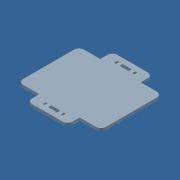
# Autodesk Inventor part: base protopress
Saved by Autodesk Inventor 2014 (Build 180170000, 170)
## iProperties
Created: 2013-09-11
Part Number: base protopress
Material: Glass
Document SubType Name: Modeling
Designer: Lefo
Density: 2.18 g/cm^3
Appearance: Clear
Author: Lefo
Autodesk Inventor part; units mm, degrees
ref_plane "YZ Plane" through (0, 0, 0) normal (1, 0, 0) x (0, 1, 0)
ref_plane "XZ Plane" through (0, 0, 0) normal (0, 1, 0) x (-1, 0, 0)
sketch "Sketch1" plane through (0, 0, 0) normal (0, 1, 0) x (-1, 0, 0)
  line L0 (0, 0) -> (-82, 0)
  line L1 (-82, 0) -> (-82, 60.3)
  line L2 (-82, 60.3) -> (0, 60.3)
  line L3 (0, 60.3) -> (0, 0)
  dimension "d0" = 82
  dimension "d1" = 60.3
  constraints: 8 end point, 2 parallel, 1 horizontal, 1 perpendicular
  measures "d0" distance of L1.end L2.end
  measures "d1" distance of L0.end L1.end
extrude "Extrusion1" add sketch "Sketch1" along normal blind 3
sketch "Sketch3" plane through (0, 3, 0) normal (0, 1, 0) x (1, 0, 0)
  line L0 (82, -60.3) -> (82, 0) projected
  line L1 (82, 0) -> (0, 0) projected
  line L2 (21, 0) -> (61, 0)
  line L3 (61, 0) -> (61, 12)
  line L4 (61, 12) -> (21, 12)
  line L5 (21, 12) -> (21, 0)
  dimension "d22" = 82
  dimension "d23" = 12
  dimension "d24" = 21
  dimension "d25" = 40
  constraints: 8 end point, 2 parallel, 1 horizontal, 1 perpendicular, 1 point on line
  measures "d22" distance of L0.end L1.end
  measures "d23" distance of L4.end L2.start
  measures "d24" distance between parallel lines of L0 L3
  measures "d25" distance of L3.end L4.end
extrude "Extrusion3" add sketch "Sketch3" against normal blind 3
sketch "Sketch4" plane through (0, 3, 0) normal (0, 1, 0) x (1, 0, 0)
  line L0 (82, 0) -> (61, 0) projected
  line L1 (61, 0) -> (61, 12) projected
  line L2 (36.5, 6.75) -> (45.5, 6.75)
  line L3 (45.5, 6.75) -> (45.5, 3.75)
  line L4 (45.5, 3.75) -> (36.5, 3.75)
  line L5 (36.5, 3.75) -> (36.5, 6.75)
  line L6 (38, 6.75) -> (43, 6.75)
  line L7 (49, 6.75) -> (51, 6.75)
  line L8 (51, 6.75) -> (51, 3.75)
  line L9 (51, 3.75) -> (49, 3.75)
  line L10 (49, 3.75) -> (49, 6.75)
  line L11 (41, 6.75) -> (41, 3.75) construction
  line L12 (33, 6.75) -> (31, 6.75)
  line L13 (31, 6.75) -> (31, 3.75)
  line L14 (31, 3.75) -> (33, 3.75)
  line L15 (33, 3.75) -> (33, 6.75)
  point P0 (21, 12)
  dimension "d28" = 9
  dimension "d29" = 3
  dimension "d30" = 3.75
  dimension "d31" = 40
  dimension "d32" = 15.5
  dimension "d42" = 2
  dimension "d43" = 3
  dimension "d44" = 3.5
  constraints: 28 end point, 4 parallel, 4 symmetric about line, 3 horizontal, 2 midpoint, 2 perpendicular, 1 collinear, 1 point on line
  measures "d28" distance of L2.start L2.end
  measures "d29" distance of L2.end L3.end
  measures "d30" distance between parallel lines of L0 L4
  measures "d31" distance of L1.end point (21, 12)
  measures "d32" distance between parallel lines of L1 L3
  measures "d42" distance of L8.end L9.end
  measures "d43" distance of L7.end L8.end
  measures "d44" distance between parallel lines of L10 L3
extrude "Extrusion4" cut sketch "Sketch4" against normal blind 3
fillet "Fillet1" radius 5 6 edges at (0, 1.5, 60.3) (82, 1.5, 60.3) (82, 1.5, 0) (61, 1.5, -12) (21, 1.5, -12) (0, 1.5, 0)
ref_plane "Work Plane1" through (5, 0, 30.15) normal (0, 0, 1) x (1, 0, 0)
mirror "Mirror1" about plane through (5, 0, 30.15) normal (0, 0, 1) of "Extrusion3", "Extrusion4"
mirror "Mirror2" about plane through (5, 0, 30.15) normal (0, 0, 1) of "Fillet1"
equation "\"d24\" = -0.5 * d25 + 0.5 * d22"
equation "\"d32\" = -0.5 * d28 + 0.5 * d31"
body "Solid1"
